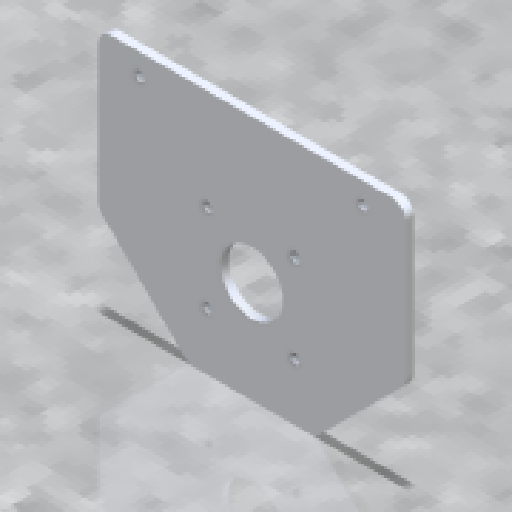
# Autodesk Inventor part: Z Axis Center Motor Mount
Saved by Autodesk Inventor 2023.2 (Build 272271000, 271)
## iProperties
Created: 2023-02-02
Part Number: Z Axis Center Motor Mount
Material: Aluminum 6061
Document SubType Name: Modeling
Designer: remop
Density: 2.7 g/cm^3
Appearance: Aluminum - Flat
Author: remop
Autodesk Inventor part; units mm, degrees
ref_plane "YZ Plane" through (0, 0, 0) normal (1, 0, 0) x (0, 1, 0)
ref_plane "XZ Plane" through (0, 0, 0) normal (0, 1, 0) x (-1, 0, 0)
ref_plane "XY Plane" through (0, 0, 0) normal (0, 0, 1) x (1, 0, 0)
sketch "Sketch1" plane through (0, 0, 0) normal (0, 0, 1) x (1, 0, 0)
  circle A0 centre (15.5, -15.5) radius 1.2295 projected
  circle A1 centre (-15.5, 15.5) radius 1.2295 projected
  circle A2 centre (-15.5, -15.5) radius 1.2295 projected
  circle A3 centre (15.5, 15.5) radius 1.2295 projected
  circle A4 centre (0, 0) radius 11 projected
  line L0 (-17.5, -21) -> (-21, -17.5) projected
  line L1 (-17.5, -21) -> (17.5, -21) projected
  line L2 (21, -17.5) -> (17.5, -21) projected
  line L3 (21, -17.5) -> (21, 17.5) projected
  line L4 (17.5, 21) -> (21, 17.5) projected
  line L5 (17.5, 21) -> (-17.5, 21) projected
  line L6 (-21, 17.5) -> (-17.5, 21) projected
  line L7 (-21, 17.5) -> (-21, -17.5) projected
  line L8 (17.5, -21) -> (22.5, -21)
  line L9 (-54.5, 51) -> (54.5, 51)
  line L10 (54.5, 51) -> (54.5, 11)
  line L11 (54.5, 11) -> (22.5, -21)
  line L12 (-17.5, -21) -> (-22.5, -21)
  line L13 (-22.5, -21) -> (-54.5, 11)
  line L14 (-54.5, 11) -> (-54.5, 51)
  circle A5 centre (-39.5, 43.5) radius 1.75
  circle A6 centre (39.5, 43.5) radius 1.75
  circle A7 centre (-15.5, 15.5) radius 1.75
  circle A8 centre (15.5, 15.5) radius 1.75
  circle A9 centre (15.5, -15.5) radius 1.75
  circle A10 centre (-15.5, -15.5) radius 1.75
  line L15 (22.5, -36) -> (-22.5, -36)
  line L16 (54.5, 11) -> (54.5, -4)
  line L17 (54.5, -4) -> (22.5, -36)
  line L18 (-22.5, -36) -> (-54.5, -4)
  line L19 (-54.5, -4) -> (-54.5, 11)
  dimension "d0" = 30
  dimension "d1" = 40
  dimension "d2" = 5
  dimension "d3" = 7.5
  dimension "d4" = 15
  dimension "d5" = 15
  dimension "d6" = 3.5
  dimension "d7" = 3.5
  dimension "d11" = 15
  constraints: 24 end point, 6 centre point, 5 parallel, 4 equal radius, 4 horizontal, 2 coincident, 2 equal length, 2 vertical, 2 vertical alignment, 1 horizontal alignment, 1 perpendicular
  measures "d0" distance between parallel lines of L5 L9
  measures "d1" distance of L13.end L9.start
  measures "d2" distance of L0.start L12.end
  measures "d3" distance from line of L9 A5.centre
  measures "d4" distance from line of L14 A5.centre
  measures "d5" distance from line of L10 A6.centre
  measures "d6" diameter of A5
  measures "d7" diameter of A7
  measures "d11" distance between parallel lines of L15 L12
extrude "Extrusion1" add sketch "Sketch1" along normal blind 3 contours L12 L13 L14 L9 L10 L11 L8 L2 L3 L4 L5 L6 L7 L0 | L0 L7 L6 L5 L4 L3 L2 L1 | L1 L8 L11 L16 L17 L15 L18 L19 L13 L12
fillet "Fillet1" radius 5 6 edges at (54.5, 51, 1.5) (-54.5, 51, 1.5) (54.5, -4, 1.5) (22.5, -36, 1.5) (-22.5, -36, 1.5) (-54.5, -4, 1.5)
equation "\"d5\" = d4"
body "Solid1"
